Autodesk Inventor part; units mm, degrees
(part 5 of 5)
  line L363 (-55.9404, 7.4643) -> (31.7396, 7.4643) projected
  arc A384 (31.7396, 7.4643) -> (34.7396, 10.4643) centre (31.7396, 10.4643) ccw projected
  line L364 (34.7396, 10.4643) -> (34.7396, 20.3443) projected
  arc A385 (34.7396, 20.3443) -> (31.7396, 23.3443) centre (31.7396, 20.3443) ccw projected
  line L365 (31.7396, 23.3443) -> (-55.9404, 23.3443) projected
  arc A386 (-55.9404, 23.3443) -> (-58.9404, 20.3443) centre (-55.9404, 20.3443) ccw projected
  circle A387 centre (16.1067, -140) radius 2.25 projected
  circle A388 centre (-17.8933, -140) radius 2.25 projected
  line L366 (-75, 46.0635) -> (-78, 46.0635) projected
  line L367 (-78, 46.0635) -> (-78, 215) projected
  line L368 (-78, 215) -> (80.4, 215) projected
  line L369 (80.4, 215) -> (80.4, 184.5) projected
  line L370 (80.4, 184.5) -> (98, 184.5) projected
  line L371 (98, 184.5) -> (98, -129) projected
  line L372 (98, -129) -> (23.6067, -129) projected
  line L373 (23.6067, -129) -> (23.6067, -146.5) projected
  line L374 (23.6067, -146.5) -> (-25.3933, -146.5) projected
  line L375 (-25.3933, -146.5) -> (-25.3933, -129) projected
  line L376 (-25.3933, -129) -> (-75, -129) projected
  line L377 (-75, -129) -> (-75, -112.7392) projected
  line L378 (-75, -112.7392) -> (-78, -112.7392) projected
  line L379 (-78, -112.7392) -> (-78, -102.4522) projected
  line L380 (-78, -102.4522) -> (-75, -102.4522) projected
  line L381 (-75, -102.4522) -> (-75, -92.3938) projected
  line L382 (-75, -92.3938) -> (-78, -92.3938) projected
  line L383 (-78, -92.3938) -> (-78, -82.1068) projected
  line L384 (-78, -82.1068) -> (-75, -82.1068) projected
  line L385 (-75, -82.1068) -> (-75, -71.7392) projected
  line L386 (-75, -71.7392) -> (-78, -71.7392) projected
  line L387 (-78, -71.7392) -> (-78, -61.4522) projected
  line L388 (-78, -61.4522) -> (-75, -61.4522) projected
  line L389 (-75, -61.4522) -> (-75, -51.3938) projected
  line L390 (-75, -51.3938) -> (-78, -51.3938) projected
  line L391 (-78, -51.3938) -> (-78, -41.1068) projected
  line L392 (-78, -41.1068) -> (-75, -41.1068) projected
  line L393 (-75, -41.1068) -> (-75, -30.7392) projected
  line L394 (-75, -30.7392) -> (-78, -30.7392) projected
  line L395 (-78, -30.7392) -> (-78, -20.4522) projected
  line L396 (-78, -20.4522) -> (-75, -20.4522) projected
  line L397 (-75, -20.4522) -> (-75, -10.3938) projected
  line L398 (-75, -10.3938) -> (-78, -10.3938) projected
  line L399 (-78, -10.3938) -> (-78, -0.1068) projected
  line L400 (-78, -0.1068) -> (-75, -0.1068) projected
  line L401 (-75, -0.1068) -> (-75, 10.2608) projected
  line L402 (-75, 10.2608) -> (-78, 10.2608) projected
  line L403 (-78, 10.2608) -> (-78, 20.5478) projected
  line L404 (-78, 20.5478) -> (-75, 20.5478) projected
  line L405 (-75, 20.5478) -> (-75, 30.6062) projected
  line L406 (-75, 30.6062) -> (-78, 30.6062) projected
  line L407 (-78, 30.6062) -> (-78, 40.8932) projected
  line L408 (-78, 40.8932) -> (-75, 40.8932) projected
  line L409 (-75, 40.8932) -> (-75, 46.0635) projected
  circle A389 centre (88, -117.6237) radius 2.25 projected
  circle A390 centre (88, 58.3987) radius 2.25 projected
  circle A391 centre (88, 131.8987) radius 2.25 projected
  circle A392 centre (88, 174.5) radius 2.25 projected
  line L410 (64, -109.7094) -> (64, 48.3987) projected
  line L411 (64, 48.3987) -> (44.819, 48.3987) projected
  arc A393 (43.3362, 49.0566) -> (44.819, 48.3987) centre (44.819, 50.3987) ccw projected
  arc A394 (43.3362, 49.0566) -> (39.7673, 49.2221) centre (41.4696, 47.3672) ccw projected
  arc A395 (39.7673, 49.2221) -> (39.1196, 47.7485) centre (41.1196, 47.7485) ccw projected
  line L412 (39.1196, 47.7485) -> (39.1196, 42.7924) projected
  arc A396 (39.1196, 42.7924) -> (39.7673, 41.3189) centre (41.1196, 42.7924) ccw projected
  arc A397 (39.7673, 41.3189) -> (39.937, 41.1764) centre (41.4696, 43.1738) ccw projected
  arc A398 (40.7196, 39.5896) -> (39.937, 41.1764) centre (38.7196, 39.5896) ccw projected
  line L413 (40.7196, 39.5896) -> (40.7196, 30.4514) projected
  arc A399 (39.937, 28.8646) -> (40.7196, 30.4514) centre (38.7196, 30.4514) ccw projected
  arc A400 (39.937, 28.8646) -> (39.7673, 28.7221) centre (41.4696, 26.8672) ccw projected
  arc A401 (39.7673, 28.7221) -> (39.1196, 27.2485) centre (41.1196, 27.2485) ccw projected
  line L414 (39.1196, 27.2485) -> (39.1196, 22.2924) projected
  arc A402 (39.1196, 22.2924) -> (39.7673, 20.8189) centre (41.1196, 22.2924) ccw projected
  arc A403 (39.7673, 20.8189) -> (39.937, 20.6764) centre (41.4696, 22.6738) ccw projected
  arc A404 (40.7196, 19.0896) -> (39.937, 20.6764) centre (38.7196, 19.0896) ccw projected
  line L415 (40.7196, 19.0896) -> (40.7196, 9.9514) projected
  arc A405 (39.937, 8.3646) -> (40.7196, 9.9514) centre (38.7196, 9.9514) ccw projected
  arc A406 (39.937, 8.3646) -> (39.7673, 8.2221) centre (41.4696, 6.3672) ccw projected
  arc A407 (39.7673, 8.2221) -> (39.1196, 6.7485) centre (41.1196, 6.7485) ccw projected
  line L416 (39.1196, 6.7485) -> (39.1196, 1.7924) projected
  arc A408 (39.1196, 1.7924) -> (39.7673, 0.3189) centre (41.1196, 1.7924) ccw projected
  arc A409 (39.7673, 0.3189) -> (39.937, 0.1764) centre (41.4696, 2.1738) ccw projected
  arc A410 (40.7196, -1.4104) -> (39.937, 0.1764) centre (38.7196, -1.4104) ccw projected
  line L417 (40.7196, -1.4104) -> (40.7196, -10.5486) projected
  arc A411 (39.937, -12.1354) -> (40.7196, -10.5486) centre (38.7196, -10.5486) ccw projected
  arc A412 (39.937, -12.1354) -> (39.7673, -12.2779) centre (41.4696, -14.1328) ccw projected
  arc A413 (39.7673, -12.2779) -> (39.1196, -13.7515) centre (41.1196, -13.7515) ccw projected
  line L418 (39.1196, -13.7515) -> (39.1196, -18.7076) projected
  arc A414 (39.1196, -18.7076) -> (39.7673, -20.1811) centre (41.1196, -18.7076) ccw projected
  arc A415 (39.7673, -20.1811) -> (39.937, -20.3236) centre (41.4696, -18.3262) ccw projected
  arc A416 (40.7196, -21.9104) -> (39.937, -20.3236) centre (38.7196, -21.9104) ccw projected
  line L419 (40.7196, -21.9104) -> (40.7196, -31.0486) projected
  arc A417 (39.937, -32.6354) -> (40.7196, -31.0486) centre (38.7196, -31.0486) ccw projected
  arc A418 (39.937, -32.6354) -> (39.7673, -32.7779) centre (41.4696, -34.6328) ccw projected
  arc A419 (39.7673, -32.7779) -> (39.1196, -34.2515) centre (41.1196, -34.2515) ccw projected
  line L420 (39.1196, -34.2515) -> (39.1196, -39.2076) projected
  arc A420 (39.1196, -39.2076) -> (39.7673, -40.6811) centre (41.1196, -39.2076) ccw projected
  arc A421 (39.7673, -40.6811) -> (39.937, -40.8236) centre (41.4696, -38.8262) ccw projected
  arc A422 (40.7196, -42.4104) -> (39.937, -40.8236) centre (38.7196, -42.4104) ccw projected
  line L421 (40.7196, -42.4104) -> (40.7196, -51.5486) projected
  arc A423 (39.937, -53.1354) -> (40.7196, -51.5486) centre (38.7196, -51.5486) ccw projected
  arc A424 (39.937, -53.1354) -> (39.7673, -53.2779) centre (41.4696, -55.1328) ccw projected
  arc A425 (39.7673, -53.2779) -> (39.1196, -54.7515) centre (41.1196, -54.7515) ccw projected
  line L422 (39.1196, -54.7515) -> (39.1196, -59.7076) projected
  arc A426 (39.1196, -59.7076) -> (39.7673, -61.1811) centre (41.1196, -59.7076) ccw projected
  arc A427 (39.7673, -61.1811) -> (39.937, -61.3236) centre (41.4696, -59.3262) ccw projected
  arc A428 (40.7196, -62.9104) -> (39.937, -61.3236) centre (38.7196, -62.9104) ccw projected
  line L423 (40.7196, -62.9104) -> (40.7196, -72.0486) projected
  arc A429 (39.937, -73.6354) -> (40.7196, -72.0486) centre (38.7196, -72.0486) ccw projected
  arc A430 (39.937, -73.6354) -> (39.7673, -73.7779) centre (41.4696, -75.6328) ccw projected
  arc A431 (39.7673, -73.7779) -> (39.1196, -75.2515) centre (41.1196, -75.2515) ccw projected
  line L424 (39.1196, -75.2515) -> (39.1196, -80.2076) projected
  arc A432 (39.1196, -80.2076) -> (39.7673, -81.6811) centre (41.1196, -80.2076) ccw projected
  arc A433 (39.7673, -81.6811) -> (39.937, -81.8236) centre (41.4696, -79.8262) ccw projected
  arc A434 (40.7196, -83.4104) -> (39.937, -81.8236) centre (38.7196, -83.4104) ccw projected
  line L425 (40.7196, -83.4104) -> (40.7196, -92.5486) projected
  arc A435 (39.937, -94.1354) -> (40.7196, -92.5486) centre (38.7196, -92.5486) ccw projected
  arc A436 (39.937, -94.1354) -> (39.7673, -94.2779) centre (41.4696, -96.1328) ccw projected
  arc A437 (39.7673, -94.2779) -> (39.1196, -95.7515) centre (41.1196, -95.7515) ccw projected
  line L426 (39.1196, -95.7515) -> (39.1196, -100.7076) projected
  arc A438 (39.1196, -100.7076) -> (39.7673, -102.1811) centre (41.1196, -100.7076) ccw projected
  arc A439 (39.7673, -102.1811) -> (40.773, -102.7455) centre (41.4696, -100.3262) ccw projected
  arc A440 (42.2196, -104.6674) -> (40.773, -102.7455) centre (40.2196, -104.6674) ccw projected
  line L427 (42.2196, -104.6674) -> (42.2196, -114.1237) projected
  arc A441 (42.2196, -114.1237) -> (43.2196, -115.1237) centre (43.2196, -114.1237) ccw projected
  line L428 (43.2196, -115.1237) -> (58.5858, -115.1237) projected
  arc A442 (58.5858, -115.1237) -> (59.2929, -114.8308) centre (58.5858, -114.1237) ccw projected
  line L429 (59.2929, -114.8308) -> (63.7071, -110.4166) projected
  arc A443 (63.7071, -110.4166) -> (64, -109.7094) centre (63, -109.7094) ccw projected
  line L430 (-69.3194, 207.0635) -> (-69.3194, 50.0635) projected
  arc A444 (-69.3194, 50.0635) -> (-68.3194, 49.0635) centre (-68.3194, 50.0635) ccw projected
  line L431 (-68.3194, 49.0635) -> (-25.6194, 49.0635) projected
  arc A445 (-25.6194, 49.0635) -> (-24.6194, 50.0635) centre (-25.6194, 50.0635) ccw projected
  line L432 (-24.6194, 50.0635) -> (-24.6194, 207.0635) projected
  arc A446 (-24.6194, 207.0635) -> (-25.6194, 208.0635) centre (-25.6194, 207.0635) ccw projected
  line L433 (-25.6194, 208.0635) -> (-68.3194, 208.0635) projected
  arc A447 (-68.3194, 208.0635) -> (-69.3194, 207.0635) centre (-68.3194, 207.0635) ccw projected
  arc A448 (31.7396, -114.6081) -> (34.7396, -111.6081) centre (31.7396, -111.6081) ccw projected
  line L434 (34.7396, -111.6081) -> (34.7396, -101.7281) projected
  arc A449 (34.7396, -101.7281) -> (31.7396, -98.7281) centre (31.7396, -101.7281) ccw projected
  line L435 (31.7396, -98.7281) -> (-55.9404, -98.7281) projected
  arc A450 (-55.9404, -98.7281) -> (-58.9404, -101.7281) centre (-55.9404, -101.7281) ccw projected
  line L436 (-58.9404, -101.7281) -> (-58.9404, -111.6081) projected
  arc A451 (-58.9404, -111.6081) -> (-55.9404, -114.6081) centre (-55.9404, -111.6081) ccw projected
  line L437 (-55.9404, -114.6081) -> (31.7396, -114.6081) projected
  arc A452 (34.7396, -81.3827) -> (31.7396, -78.3827) centre (31.7396, -81.3827) ccw projected
  line L438 (31.7396, -78.3827) -> (-55.9404, -78.3827) projected
  arc A453 (-55.9404, -78.3827) -> (-58.9404, -81.3827) centre (-55.9404, -81.3827) ccw projected
  line L439 (-58.9404, -81.3827) -> (-58.9404, -91.2627) projected
  arc A454 (-58.9404, -91.2627) -> (-55.9404, -94.2627) centre (-55.9404, -91.2627) ccw projected
  line L440 (-55.9404, -94.2627) -> (31.7396, -94.2627) projected
  arc A455 (31.7396, -94.2627) -> (34.7396, -91.2627) centre (31.7396, -91.2627) ccw projected
  line L441 (34.7396, -91.2627) -> (34.7396, -81.3827) projected
  line L442 (-55.9404, -33.2265) -> (31.7396, -33.2265) projected
  arc A456 (31.7396, -33.2265) -> (34.7396, -30.2265) centre (31.7396, -30.2265) ccw projected
  line L443 (34.7396, -30.2265) -> (34.7396, -20.3465) projected
  arc A457 (34.7396, -20.3465) -> (31.7396, -17.3465) centre (31.7396, -20.3465) ccw projected
  line L444 (31.7396, -17.3465) -> (-55.9404, -17.3465) projected
  arc A458 (-55.9404, -17.3465) -> (-58.9404, -20.3465) centre (-55.9404, -20.3465) ccw projected
  line L445 (-58.9404, -20.3465) -> (-58.9404, -30.2265) projected
  arc A459 (-58.9404, -30.2265) -> (-55.9404, -33.2265) centre (-55.9404, -30.2265) ccw projected
  line L446 (31.7396, -58.0373) -> (-55.9404, -58.0373) projected
  arc A460 (-55.9404, -58.0373) -> (-58.9404, -61.0373) centre (-55.9404, -61.0373) ccw projected
  line L447 (-58.9404, -61.0373) -> (-58.9404, -70.9173) projected
  arc A461 (-58.9404, -70.9173) -> (-55.9404, -73.9173) centre (-55.9404, -70.9173) ccw projected
  line L448 (-55.9404, -73.9173) -> (31.7396, -73.9173) projected
  arc A462 (31.7396, -73.9173) -> (34.7396, -70.9173) centre (31.7396, -70.9173) ccw projected
  line L449 (34.7396, -70.9173) -> (34.7396, -61.0373) projected
  arc A463 (34.7396, -61.0373) -> (31.7396, -58.0373) centre (31.7396, -61.0373) ccw projected
  arc A464 (-55.9404, -37.6919) -> (-58.9404, -40.6919) centre (-55.9404, -40.6919) ccw projected
  line L450 (-58.9404, -40.6919) -> (-58.9404, -50.5719) projected
  arc A465 (-58.9404, -50.5719) -> (-55.9404, -53.5719) centre (-55.9404, -50.5719) ccw projected
  line L451 (-55.9404, -53.5719) -> (31.7396, -53.5719) projected
  arc A466 (31.7396, -53.5719) -> (34.7396, -50.5719) centre (31.7396, -50.5719) ccw projected
  line L452 (34.7396, -50.5719) -> (34.7396, -40.6919) projected
  arc A467 (34.7396, -40.6919) -> (31.7396, -37.6919) centre (31.7396, -40.6919) ccw projected
  line L453 (31.7396, -37.6919) -> (-55.9404, -37.6919) projected
  arc A468 (-55.9404, 2.9989) -> (-58.9404, -0.0011) centre (-55.9404, -0.0011) ccw projected
  line L454 (-58.9404, -0.0011) -> (-58.9404, -9.8811) projected
  arc A469 (-58.9404, -9.8811) -> (-55.9404, -12.8811) centre (-55.9404, -9.8811) ccw projected
  line L455 (-55.9404, -12.8811) -> (31.7396, -12.8811) projected
  arc A470 (31.7396, -12.8811) -> (34.7396, -9.8811) centre (31.7396, -9.8811) ccw projected
  line L456 (34.7396, -9.8811) -> (34.7396, -0.0011) projected
  arc A471 (34.7396, -0.0011) -> (31.7396, 2.9989) centre (31.7396, -0.0011) ccw projected
  line L457 (31.7396, 2.9989) -> (-55.9404, 2.9989) projected
  line L458 (-58.9404, 40.6897) -> (-58.9404, 30.8097) projected
  arc A472 (-58.9404, 30.8097) -> (-55.9404, 27.8097) centre (-55.9404, 30.8097) ccw projected
  line L459 (-55.9404, 27.8097) -> (31.7396, 27.8097) projected
  arc A473 (31.7396, 27.8097) -> (34.7396, 30.8097) centre (31.7396, 30.8097) ccw projected
  line L460 (34.7396, 30.8097) -> (34.7396, 40.6897) projected
  arc A474 (34.7396, 40.6897) -> (31.7396, 43.6897) centre (31.7396, 40.6897) ccw projected
  line L461 (31.7396, 43.6897) -> (-55.9404, 43.6897) projected
  arc A475 (-55.9404, 43.6897) -> (-58.9404, 40.6897) centre (-55.9404, 40.6897) ccw projected
  line L462 (-58.9404, 20.3443) -> (-58.9404, 10.4643) projected
  arc A476 (-58.9404, 10.4643) -> (-55.9404, 7.4643) centre (-55.9404, 10.4643) ccw projected
  line L463 (-55.9404, 7.4643) -> (31.7396, 7.4643) projected
  arc A477 (31.7396, 7.4643) -> (34.7396, 10.4643) centre (31.7396, 10.4643) ccw projected
  line L464 (34.7396, 10.4643) -> (34.7396, 20.3443) projected
  arc A478 (34.7396, 20.3443) -> (31.7396, 23.3443) centre (31.7396, 20.3443) ccw projected
  line L465 (31.7396, 23.3443) -> (-55.9404, 23.3443) projected
  arc A479 (-55.9404, 23.3443) -> (-58.9404, 20.3443) centre (-55.9404, 20.3443) ccw projected
  circle A480 centre (16.1067, -140) radius 2.25 projected
  circle A481 centre (-17.8933, -140) radius 2.25 projected
  line L466 (-75, 46.0635) -> (-78, 46.0635) projected
  line L467 (-78, 46.0635) -> (-78, 215) projected
  line L468 (-78, 215) -> (80.4, 215) projected
  line L469 (80.4, 215) -> (80.4, 184.5) projected
  line L470 (80.4, 184.5) -> (98, 184.5) projected
  line L471 (98, 184.5) -> (98, -129) projected
  line L472 (98, -129) -> (23.6067, -129) projected
  line L473 (23.6067, -129) -> (23.6067, -146.5) projected
  line L474 (23.6067, -146.5) -> (-25.3933, -146.5) projected
  line L475 (-25.3933, -146.5) -> (-25.3933, -129) projected
  line L476 (-25.3933, -129) -> (-75, -129) projected
  line L477 (-75, -129) -> (-75, -112.7392) projected
  line L478 (-75, -112.7392) -> (-78, -112.7392) projected
  line L479 (-78, -112.7392) -> (-78, -102.4522) projected
  line L480 (-78, -102.4522) -> (-75, -102.4522) projected
  line L481 (-75, -102.4522) -> (-75, -92.3938) projected
  line L482 (-75, -92.3938) -> (-78, -92.3938) projected
  line L483 (-78, -92.3938) -> (-78, -82.1068) projected
  line L484 (-78, -82.1068) -> (-75, -82.1068) projected
  line L485 (-75, -82.1068) -> (-75, -71.7392) projected
  line L486 (-75, -71.7392) -> (-78, -71.7392) projected
  line L487 (-78, -71.7392) -> (-78, -61.4522) projected
  line L488 (-78, -61.4522) -> (-75, -61.4522) projected
  line L489 (-75, -61.4522) -> (-75, -51.3938) projected
  line L490 (-75, -51.3938) -> (-78, -51.3938) projected
  line L491 (-78, -51.3938) -> (-78, -41.1068) projected
  line L492 (-78, -41.1068) -> (-75, -41.1068) projected
  line L493 (-75, -41.1068) -> (-75, -30.7392) projected
  line L494 (-75, -30.7392) -> (-78, -30.7392) projected
  line L495 (-78, -30.7392) -> (-78, -20.4522) projected
  line L496 (-78, -20.4522) -> (-75, -20.4522) projected
  line L497 (-75, -20.4522) -> (-75, -10.3938) projected
  line L498 (-75, -10.3938) -> (-78, -10.3938) projected
  line L499 (-78, -10.3938) -> (-78, -0.1068) projected
  line L500 (-78, -0.1068) -> (-75, -0.1068) projected
  line L501 (-75, -0.1068) -> (-75, 10.2608) projected
  line L502 (-75, 10.2608) -> (-78, 10.2608) projected
  line L503 (-78, 10.2608) -> (-78, 20.5478) projected
  line L504 (-78, 20.5478) -> (-75, 20.5478) projected
  line L505 (-75, 20.5478) -> (-75, 30.6062) projected
  line L506 (-75, 30.6062) -> (-78, 30.6062) projected
  line L507 (-78, 30.6062) -> (-78, 40.8932) projected
  line L508 (-78, 40.8932) -> (-75, 40.8932) projected
  line L509 (-75, 40.8932) -> (-75, 46.0635) projected
  circle A482 centre (88, -117.6237) radius 2.25 projected
  circle A483 centre (88, 58.3987) radius 2.25 projected
  circle A484 centre (88, 131.8987) radius 2.25 projected
  circle A485 centre (88, 174.5) radius 2.25 projected
  line L510 (64, -109.7094) -> (64, 48.3987) projected
  line L511 (64, 48.3987) -> (44.819, 48.3987) projected
  arc A486 (43.3362, 49.0566) -> (44.819, 48.3987) centre (44.819, 50.3987) ccw projected
  arc A487 (43.3362, 49.0566) -> (39.7673, 49.2221) centre (41.4696, 47.3672) ccw projected
  arc A488 (39.7673, 49.2221) -> (39.1196, 47.7485) centre (41.1196, 47.7485) ccw projected
  line L512 (39.1196, 47.7485) -> (39.1196, 42.7924) projected
  arc A489 (39.1196, 42.7924) -> (39.7673, 41.3189) centre (41.1196, 42.7924) ccw projected
  arc A490 (39.7673, 41.3189) -> (39.937, 41.1764) centre (41.4696, 43.1738) ccw projected
  arc A491 (40.7196, 39.5896) -> (39.937, 41.1764) centre (38.7196, 39.5896) ccw projected
  line L513 (40.7196, 39.5896) -> (40.7196, 30.4514) projected
  arc A492 (39.937, 28.8646) -> (40.7196, 30.4514) centre (38.7196, 30.4514) ccw projected
  arc A493 (39.937, 28.8646) -> (39.7673, 28.7221) centre (41.4696, 26.8672) ccw projected
  arc A494 (39.7673, 28.7221) -> (39.1196, 27.2485) centre (41.1196, 27.2485) ccw projected
  line L514 (39.1196, 27.2485) -> (39.1196, 22.2924) projected
  arc A495 (39.1196, 22.2924) -> (39.7673, 20.8189) centre (41.1196, 22.2924) ccw projected
  arc A496 (39.7673, 20.8189) -> (39.937, 20.6764) centre (41.4696, 22.6738) ccw projected
  arc A497 (40.7196, 19.0896) -> (39.937, 20.6764) centre (38.7196, 19.0896) ccw projected
  line L515 (40.7196, 19.0896) -> (40.7196, 9.9514) projected
  arc A498 (39.937, 8.3646) -> (40.7196, 9.9514) centre (38.7196, 9.9514) ccw projected
  arc A499 (39.937, 8.3646) -> (39.7673, 8.2221) centre (41.4696, 6.3672) ccw projected
  arc A500 (39.7673, 8.2221) -> (39.1196, 6.7485) centre (41.1196, 6.7485) ccw projected
  line L516 (39.1196, 6.7485) -> (39.1196, 1.7924) projected
  arc A501 (39.1196, 1.7924) -> (39.7673, 0.3189) centre (41.1196, 1.7924) ccw projected
  arc A502 (39.7673, 0.3189) -> (39.937, 0.1764) centre (41.4696, 2.1738) ccw projected
  arc A503 (40.7196, -1.4104) -> (39.937, 0.1764) centre (38.7196, -1.4104) ccw projected
  line L517 (40.7196, -1.4104) -> (40.7196, -10.5486) projected
  arc A504 (39.937, -12.1354) -> (40.7196, -10.5486) centre (38.7196, -10.5486) ccw projected
  arc A505 (39.937, -12.1354) -> (39.7673, -12.2779) centre (41.4696, -14.1328) ccw projected
  arc A506 (39.7673, -12.2779) -> (39.1196, -13.7515) centre (41.1196, -13.7515) ccw projected
  line L518 (39.1196, -13.7515) -> (39.1196, -18.7076) projected
  arc A507 (39.1196, -18.7076) -> (39.7673, -20.1811) centre (41.1196, -18.7076) ccw projected
  arc A508 (39.7673, -20.1811) -> (39.937, -20.3236) centre (41.4696, -18.3262) ccw projected
  arc A509 (40.7196, -21.9104) -> (39.937, -20.3236) centre (38.7196, -21.9104) ccw projected
  line L519 (40.7196, -21.9104) -> (40.7196, -31.0486) projected
  arc A510 (39.937, -32.6354) -> (40.7196, -31.0486) centre (38.7196, -31.0486) ccw projected
  arc A511 (39.937, -32.6354) -> (39.7673, -32.7779) centre (41.4696, -34.6328) ccw projected
  arc A512 (39.7673, -32.7779) -> (39.1196, -34.2515) centre (41.1196, -34.2515) ccw projected
  line L520 (39.1196, -34.2515) -> (39.1196, -39.2076) projected
  arc A513 (39.1196, -39.2076) -> (39.7673, -40.6811) centre (41.1196, -39.2076) ccw projected
  arc A514 (39.7673, -40.6811) -> (39.937, -40.8236) centre (41.4696, -38.8262) ccw projected
  arc A515 (40.7196, -42.4104) -> (39.937, -40.8236) centre (38.7196, -42.4104) ccw projected
  line L521 (40.7196, -42.4104) -> (40.7196, -51.5486) projected
  arc A516 (39.937, -53.1354) -> (40.7196, -51.5486) centre (38.7196, -51.5486) ccw projected
  arc A517 (39.937, -53.1354) -> (39.7673, -53.2779) centre (41.4696, -55.1328) ccw projected
  arc A518 (39.7673, -53.2779) -> (39.1196, -54.7515) centre (41.1196, -54.7515) ccw projected
  line L522 (39.1196, -54.7515) -> (39.1196, -59.7076) projected
  arc A519 (39.1196, -59.7076) -> (39.7673, -61.1811) centre (41.1196, -59.7076) ccw projected
  arc A520 (39.7673, -61.1811) -> (39.937, -61.3236) centre (41.4696, -59.3262) ccw projected
  arc A521 (40.7196, -62.9104) -> (39.937, -61.3236) centre (38.7196, -62.9104) ccw projected
  line L523 (40.7196, -62.9104) -> (40.7196, -72.0486) projected
  arc A522 (39.937, -73.6354) -> (40.7196, -72.0486) centre (38.7196, -72.0486) ccw projected
  arc A523 (39.937, -73.6354) -> (39.7673, -73.7779) centre (41.4696, -75.6328) ccw projected
  arc A524 (39.7673, -73.7779) -> (39.1196, -75.2515) centre (41.1196, -75.2515) ccw projected
  line L524 (39.1196, -75.2515) -> (39.1196, -80.2076) projected
  arc A525 (39.1196, -80.2076) -> (39.7673, -81.6811) centre (41.1196, -80.2076) ccw projected
  arc A526 (39.7673, -81.6811) -> (39.937, -81.8236) centre (41.4696, -79.8262) ccw projected
  arc A527 (40.7196, -83.4104) -> (39.937, -81.8236) centre (38.7196, -83.4104) ccw projected
  line L525 (40.7196, -83.4104) -> (40.7196, -92.5486) projected
  arc A528 (39.937, -94.1354) -> (40.7196, -92.5486) centre (38.7196, -92.5486) ccw projected
  arc A529 (39.937, -94.1354) -> (39.7673, -94.2779) centre (41.4696, -96.1328) ccw projected
  arc A530 (39.7673, -94.2779) -> (39.1196, -95.7515) centre (41.1196, -95.7515) ccw projected
  line L526 (39.1196, -95.7515) -> (39.1196, -100.7076) projected
  arc A531 (39.1196, -100.7076) -> (39.7673, -102.1811) centre (41.1196, -100.7076) ccw projected
  arc A532 (39.7673, -102.1811) -> (40.773, -102.7455) centre (41.4696, -100.3262) ccw projected
  arc A533 (42.2196, -104.6674) -> (40.773, -102.7455) centre (40.2196, -104.6674) ccw projected
  line L527 (42.2196, -104.6674) -> (42.2196, -114.1237) projected
  arc A534 (42.2196, -114.1237) -> (43.2196, -115.1237) centre (43.2196, -114.1237) ccw projected
  line L528 (43.2196, -115.1237) -> (58.5858, -115.1237) projected
  arc A535 (58.5858, -115.1237) -> (59.2929, -114.8308) centre (58.5858, -114.1237) ccw projected
  line L529 (59.2929, -114.8308) -> (63.7071, -110.4166) projected
  arc A536 (63.7071, -110.4166) -> (64, -109.7094) centre (63, -109.7094) ccw projected
  line L530 (-69.3194, 207.0635) -> (-69.3194, 50.0635) projected
  arc A537 (-69.3194, 50.0635) -> (-68.3194, 49.0635) centre (-68.3194, 50.0635) ccw projected
  line L531 (-68.3194, 49.0635) -> (-25.6194, 49.0635) projected
  arc A538 (-25.6194, 49.0635) -> (-24.6194, 50.0635) centre (-25.6194, 50.0635) ccw projected
  line L532 (-24.6194, 50.0635) -> (-24.6194, 207.0635) projected
  arc A539 (-24.6194, 207.0635) -> (-25.6194, 208.0635) centre (-25.6194, 207.0635) ccw projected
  line L533 (-25.6194, 208.0635) -> (-68.3194, 208.0635) projected
  arc A540 (-68.3194, 208.0635) -> (-69.3194, 207.0635) centre (-68.3194, 207.0635) ccw projected
  arc A541 (31.7396, -114.6081) -> (34.7396, -111.6081) centre (31.7396, -111.6081) ccw projected
  line L534 (34.7396, -111.6081) -> (34.7396, -101.7281) projected
  arc A542 (34.7396, -101.7281) -> (31.7396, -98.7281) centre (31.7396, -101.7281) ccw projected
  line L535 (31.7396, -98.7281) -> (-55.9404, -98.7281) projected
  arc A543 (-55.9404, -98.7281) -> (-58.9404, -101.7281) centre (-55.9404, -101.7281) ccw projected
  line L536 (-58.9404, -101.7281) -> (-58.9404, -111.6081) projected
  arc A544 (-58.9404, -111.6081) -> (-55.9404, -114.6081) centre (-55.9404, -111.6081) ccw projected
  line L537 (-55.9404, -114.6081) -> (31.7396, -114.6081) projected
  arc A545 (34.7396, -81.3827) -> (31.7396, -78.3827) centre (31.7396, -81.3827) ccw projected
  line L538 (31.7396, -78.3827) -> (-55.9404, -78.3827) projected
  arc A546 (-55.9404, -78.3827) -> (-58.9404, -81.3827) centre (-55.9404, -81.3827) ccw projected
  line L539 (-58.9404, -81.3827) -> (-58.9404, -91.2627) projected
  arc A547 (-58.9404, -91.2627) -> (-55.9404, -94.2627) centre (-55.9404, -91.2627) ccw projected
  line L540 (-55.9404, -94.2627) -> (31.7396, -94.2627) projected
  arc A548 (31.7396, -94.2627) -> (34.7396, -91.2627) centre (31.7396, -91.2627) ccw projected
  line L541 (34.7396, -91.2627) -> (34.7396, -81.3827) projected
  line L542 (-55.9404, -33.2265) -> (31.7396, -33.2265) projected
  arc A549 (31.7396, -33.2265) -> (34.7396, -30.2265) centre (31.7396, -30.2265) ccw projected
  line L543 (34.7396, -30.2265) -> (34.7396, -20.3465) projected
  arc A550 (34.7396, -20.3465) -> (31.7396, -17.3465) centre (31.7396, -20.3465) ccw projected
  line L544 (31.7396, -17.3465) -> (-55.9404, -17.3465) projected
  arc A551 (-55.9404, -17.3465) -> (-58.9404, -20.3465) centre (-55.9404, -20.3465) ccw projected
  line L545 (-58.9404, -20.3465) -> (-58.9404, -30.2265) projected
  arc A552 (-58.9404, -30.2265) -> (-55.9404, -33.2265) centre (-55.9404, -30.2265) ccw projected
  line L546 (31.7396, -58.0373) -> (-55.9404, -58.0373) projected
  arc A553 (-55.9404, -58.0373) -> (-58.9404, -61.0373) centre (-55.9404, -61.0373) ccw projected
  line L547 (-58.9404, -61.0373) -> (-58.9404, -70.9173) projected
  arc A554 (-58.9404, -70.9173) -> (-55.9404, -73.9173) centre (-55.9404, -70.9173) ccw projected
  line L548 (-55.9404, -73.9173) -> (31.7396, -73.9173) projected
  arc A555 (31.7396, -73.9173) -> (34.7396, -70.9173) centre (31.7396, -70.9173) ccw projected
  line L549 (34.7396, -70.9173) -> (34.7396, -61.0373) projected
  arc A556 (34.7396, -61.0373) -> (31.7396, -58.0373) centre (31.7396, -61.0373) ccw projected
  arc A557 (-55.9404, -37.6919) -> (-58.9404, -40.6919) centre (-55.9404, -40.6919) ccw projected
  line L550 (-58.9404, -40.6919) -> (-58.9404, -50.5719) projected
  arc A558 (-58.9404, -50.5719) -> (-55.9404, -53.5719) centre (-55.9404, -50.5719) ccw projected
  line L551 (-55.9404, -53.5719) -> (31.7396, -53.5719) projected
  arc A559 (31.7396, -53.5719) -> (34.7396, -50.5719) centre (31.7396, -50.5719) ccw projected
  line L552 (34.7396, -50.5719) -> (34.7396, -40.6919) projected
  arc A560 (34.7396, -40.6919) -> (31.7396, -37.6919) centre (31.7396, -40.6919) ccw projected
  line L553 (31.7396, -37.6919) -> (-55.9404, -37.6919) projected
  arc A561 (-55.9404, 2.9989) -> (-58.9404, -0.0011) centre (-55.9404, -0.0011) ccw projected
  line L554 (-58.9404, -0.0011) -> (-58.9404, -9.8811) projected
  arc A562 (-58.9404, -9.8811) -> (-55.9404, -12.8811) centre (-55.9404, -9.8811) ccw projected
  line L555 (-55.9404, -12.8811) -> (31.7396, -12.8811) projected
  arc A563 (31.7396, -12.8811) -> (34.7396, -9.8811) centre (31.7396, -9.8811) ccw projected
  line L556 (34.7396, -9.8811) -> (34.7396, -0.0011) projected
  arc A564 (34.7396, -0.0011) -> (31.7396, 2.9989) centre (31.7396, -0.0011) ccw projected
  line L557 (31.7396, 2.9989) -> (-55.9404, 2.9989) projected
  line L558 (-58.9404, 40.6897) -> (-58.9404, 30.8097) projected
  arc A565 (-58.9404, 30.8097) -> (-55.9404, 27.8097) centre (-55.9404, 30.8097) ccw projected
  line L559 (-55.9404, 27.8097) -> (31.7396, 27.8097) projected
  arc A566 (31.7396, 27.8097) -> (34.7396, 30.8097) centre (31.7396, 30.8097) ccw projected
  line L560 (34.7396, 30.8097) -> (34.7396, 40.6897) projected
  arc A567 (34.7396, 40.6897) -> (31.7396, 43.6897) centre (31.7396, 40.6897) ccw projected
  line L561 (31.7396, 43.6897) -> (-55.9404, 43.6897) projected
  arc A568 (-55.9404, 43.6897) -> (-58.9404, 40.6897) centre (-55.9404, 40.6897) ccw projected
  line L562 (-58.9404, 20.3443) -> (-58.9404, 10.4643) projected
  arc A569 (-58.9404, 10.4643) -> (-55.9404, 7.4643) centre (-55.9404, 10.4643) ccw projected
  line L563 (-55.9404, 7.4643) -> (31.7396, 7.4643) projected
  arc A570 (31.7396, 7.4643) -> (34.7396, 10.4643) centre (31.7396, 10.4643) ccw projected
  line L564 (34.7396, 10.4643) -> (34.7396, 20.3443) projected
  arc A571 (34.7396, 20.3443) -> (31.7396, 23.3443) centre (31.7396, 20.3443) ccw projected
  line L565 (31.7396, 23.3443) -> (-55.9404, 23.3443) projected
  arc A572 (-55.9404, 23.3443) -> (-58.9404, 20.3443) centre (-55.9404, 20.3443) ccw projected
  circle A573 centre (16.1067, -140) radius 2.25 projected
  circle A574 centre (-17.8933, -140) radius 2.25 projected
  line L566 (-75, 46.0635) -> (-78, 46.0635) projected
  line L567 (-78, 46.0635) -> (-78, 215) projected
  line L568 (-78, 215) -> (80.4, 215) projected
  line L569 (80.4, 215) -> (80.4, 184.5) projected
  line L570 (80.4, 184.5) -> (98, 184.5) projected
  line L571 (98, 184.5) -> (98, -129) projected
  line L572 (98, -129) -> (23.6067, -129) projected
  line L573 (23.6067, -129) -> (23.6067, -146.5) projected
  line L574 (23.6067, -146.5) -> (-25.3933, -146.5) projected
  line L575 (-25.3933, -146.5) -> (-25.3933, -129) projected
  line L576 (-25.3933, -129) -> (-75, -129) projected
  line L577 (-75, -129) -> (-75, -112.7392) projected
  line L578 (-75, -112.7392) -> (-78, -112.7392) projected
  line L579 (-78, -112.7392) -> (-78, -102.4522) projected
  line L580 (-78, -102.4522) -> (-75, -102.4522) projected
  line L581 (-75, -102.4522) -> (-75, -92.3938) projected
  line L582 (-75, -92.3938) -> (-78, -92.3938) projected
  line L583 (-78, -92.3938) -> (-78, -82.1068) projected
  line L584 (-78, -82.1068) -> (-75, -82.1068) projected
  line L585 (-75, -82.1068) -> (-75, -71.7392) projected
  line L586 (-75, -71.7392) -> (-78, -71.7392) projected
  line L587 (-78, -71.7392) -> (-78, -61.4522) projected
  line L588 (-78, -61.4522) -> (-75, -61.4522) projected
  line L589 (-75, -61.4522) -> (-75, -51.3938) projected
  line L590 (-75, -51.3938) -> (-78, -51.3938) projected
  line L591 (-78, -51.3938) -> (-78, -41.1068) projected
  line L592 (-78, -41.1068) -> (-75, -41.1068) projected
  line L593 (-75, -41.1068) -> (-75, -30.7392) projected
  line L594 (-75, -30.7392) -> (-78, -30.7392) projected
  line L595 (-78, -30.7392) -> (-78, -20.4522) projected
  line L596 (-78, -20.4522) -> (-75, -20.4522) projected
  line L597 (-75, -20.4522) -> (-75, -10.3938) projected
  line L598 (-75, -10.3938) -> (-78, -10.3938) projected
  line L599 (-78, -10.3938) -> (-78, -0.1068) projected
  line L600 (-78, -0.1068) -> (-75, -0.1068) projected
  line L601 (-75, -0.1068) -> (-75, 10.2608) projected
  line L602 (-75, 10.2608) -> (-78, 10.2608) projected
  line L603 (-78, 10.2608) -> (-78, 20.5478) projected
  line L604 (-78, 20.5478) -> (-75, 20.5478) projected
  line L605 (-75, 20.5478) -> (-75, 30.6062) projected
  line L606 (-75, 30.6062) -> (-78, 30.6062) projected
  line L607 (-78, 30.6062) -> (-78, 40.8932) projected
  line L608 (-78, 40.8932) -> (-75, 40.8932) projected
  line L609 (-75, 40.8932) -> (-75, 46.0635) projected
  arc A575 (58.1119, 81.5843) -> (63.8901, 95.6469) centre (43.8901, 95.6462) ccw
  arc A576 (40.2515, 72.6659) -> (51.24, 75.9547) centre (40.252, 92.666) ccw
  arc A577 (51.24, 75.9547) -> (58.1119, 81.5843) centre (27.8907, 111.4659) ccw
  arc A578 (51.3434, 146.9089) -> (51.1375, 147.0443) centre (27.8907, 111.4659) ccw
  arc A579 (4.5403, 146.9769) -> (4.5403, 146.9769) centre (27.8907, 111.4659) ccw
  arc A580 (4.5403, 75.9549) -> (4.5403, 75.9549) centre (27.8907, 111.4659) ccw
  arc A581 (31.6537, 111.4659) -> (58.057, 141.4032) centre (43.8901, 127.2859) ccw
  arc A582 (51.3278, 146.9192) -> (29.485, 113.4117) centre (40.2523, 130.2659) ccw
  arc A583 (-2.4189, 81.6736) -> (4.6435, 75.8875) centre (27.8907, 111.4659) ccw
  arc A584 (58.1663, 141.2926) -> (51.205, 147.0003) centre (27.8907, 111.4659) ccw
  arc A585 (4.6435, 147.0442) -> (-2.4189, 141.2582) centre (27.8907, 111.4659) ccw
  point P0 (0, 0)
  point P1 (27.8903, 195.073)
  point P2 (15.5287, 150.2659)
  point P3 (51.2759, 146.9537)
  point P4 (51.1528, 147.0343)
  dimension "d99" = 27.2
  dimension "d100" = 19.2
  dimension "d102" = 3
  dimension "d103" = 3
  dimension "d104" = 13.6
  dimension "d105" = 9.6
  dimension "d106" = 3.5
  dimension "d107" = 20
  dimension "d108" = 3.5
  dimension "d109" = 20
  dimension "d110" = 9.6
  dimension "d111" = 9.6
  dimension "d112" = 105.0194
  dimension "d119" = 20
  dimension "d121" = 15.819
  dimension "d123" = 20
  dimension "d126" = 12.362
  dimension "d129" = 72
  dimension "d130" = 77.6
  dimension "d131" = 35.7
  dimension "d132" = 35.7
  dimension "d133" = 2.4
  dimension "d137" = 40
  dimension "d138" = 40
  constraints: 59 point on circle, 28 centre point, 20 coincident, 20 end point, 16 symmetric about line, 13 tangent, 4 parallel, 3 horizontal, 2 equal radius, 2 perpendicular, 1 point on line, 1 vertical, 6 other
  measures "d99" distance between parallel lines of L101 L103
  measures "d100" distance between parallel lines of L102 L100
  measures "d102" radius of A93
  measures "d103" radius of A94
  measures "d104" distance from line of L101 point (27.89, 195.073)
  measures "d105" distance from line of L102 point (27.89, 195.073)
  measures "d106" diameter of A97
  measures "d107" distance of point (27.89, 195.073) A97.centre
  measures "d108" diameter of A98
  measures "d109" distance of point (27.89, 195.073) A98.centre
  measures "d110" distance from line of L102 A97.centre
  measures "d111" distance from line of L102 A98.centre
  measures "d112" distance between parallel lines of L6 L78
  measures "d119" distance from line of L106 point (11.89, 95.647)
  measures "d121" vertical distance of point (27.891, 111.466) point (11.89, 95.647)
  measures "d123" distance from line of L104 point (15.529, 92.666)
  measures "d126" horizontal distance of A101.centre point (15.529, 92.666)
  measures "d129" distance between parallel lines of L109 L106
  measures "d130" distance between parallel lines of L104 L105
  measures "d131" horizontal distance of point (27.891, 111.466) point (-7.809, 75.766)
  measures "d132" horizontal distance of point (27.891, 111.466) point (-7.809, 75.766)
  measures "d133" diameter of A106
  measures "d137" diameter of A581
  measures "d138" diameter of A582
extrude "Extrusion13" cut sketch "Sketch12" against normal up to surface (3 mm away) contours A96 L103 A95 L102 A94 L101 A93 L100 | A97 | A98 | A100 A101 A99 L106 A102 A104 A103 L105 A582 L107 L108 A581 L109 A575 A577 A576 L104 | A581 L108 L107 A582 A578 A579 | A106 | A107 | A108 | A109
equation "\"d20\" = d19"
equation "\"d27\" = d26"
equation "\"d28\" = d23"
equation "\"d29\" = d24"
equation "\"d42\" = d41"
equation "\"d43\" = d40"
equation "\"d50\" = d48"
equation "\"d51\" = d49"
equation "\"d52\" = d50"
equation "\"d54\" = d52"
body "Solid2"
